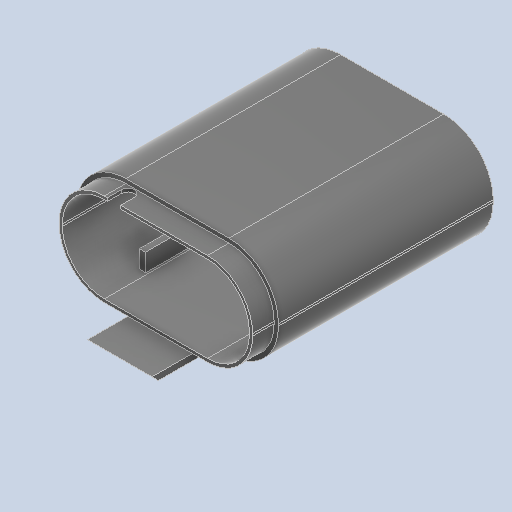
# Autodesk Inventor part: fullback
Saved by Autodesk Inventor 2024 (Build 280153000, 153)
## iProperties
Created: 2023-10-23
Part Number: fullback
Material: Acetal Resin, Black
Document SubType Name: Modeling
Designer: User Account
Density: 1.425 g/cm^3
Appearance: Smooth - Black
Author: User Account
Autodesk Inventor part; units mm, degrees
ref_plane "YZ Plane" through (0, 0, 0) normal (1, 0, 0) x (0, 1, 0)
ref_plane "XZ Plane" through (0, 0, 0) normal (0, 1, 0) x (-1, 0, 0)
ref_plane "XY Plane" through (0, 0, 0) normal (0, 0, 1) x (1, 0, 0)
sketch "Sketch1" plane through (0, 0, 0) normal (0, 0, 1) x (1, 0, 0)
  line L0 (71.0137, 43.5924) -> (23.0137, 43.5924)
  line L1 (23.0137, 41.5924) -> (71.0137, 41.5924)
  line L2 (71.0137, -1.4076) -> (23.0137, -1.4076)
  line L3 (23.0137, -3.4076) -> (71.0137, -3.4076)
  line L4 (2.0137, 19.5924) -> (2.0137, 20.5924)
  arc A0 (23.0137, 41.5924) -> (2.0137, 20.5924) centre (23.0137, 20.5924) ccw
  arc A1 (2.0137, 19.5924) -> (23.0137, -1.4076) centre (23.0137, 19.5924) ccw
  arc A2 (23.0137, 43.5924) -> (0.0137, 20.5924) centre (23.0137, 20.5924) ccw
  line L5 (0.0137, 20.5924) -> (0.0137, 19.5924)
  arc A3 (0.0137, 19.5924) -> (23.0137, -3.4076) centre (23.0137, 19.5924) ccw
  arc A4 (71.0137, -1.4076) -> (92.0137, 19.5924) centre (71.0137, 19.5924) ccw
  arc A5 (71.0137, -3.4076) -> (94.0137, 19.5924) centre (71.0137, 19.5924) ccw
  line L6 (92.0137, 20.5924) -> (92.0137, 19.5924)
  line L7 (94.0137, 19.5924) -> (94.0137, 20.5924)
  arc A6 (92.0137, 20.5924) -> (71.0137, 41.5924) centre (71.0137, 20.5924) ccw
  arc A7 (94.0137, 20.5924) -> (71.0137, 43.5924) centre (71.0137, 20.5924) ccw
  line L8 (71.0137, 40.0924) -> (23.0137, 40.0924)
  arc A8 (23.0137, 40.0924) -> (3.5137, 20.5924) centre (23.0137, 20.5924) ccw
  line L9 (3.5137, 20.5924) -> (3.5137, 19.5924)
  arc A9 (3.5137, 19.5924) -> (23.0137, 0.0924) centre (23.0137, 19.5924) ccw
  line L10 (23.0137, 0.0924) -> (71.0137, 0.0924)
  arc A10 (71.0137, 0.0924) -> (90.5137, 19.5924) centre (71.0137, 19.5924) ccw
  line L11 (90.5137, 19.5924) -> (90.5137, 20.5924)
  arc A11 (90.5137, 20.5924) -> (71.0137, 40.0924) centre (71.0137, 20.5924) ccw
  line L12 (74.7637, 0.4563) -> (74.7637, 8.4563)
  line L13 (19.2637, 8.4563) -> (19.2637, 0.4563)
  line L14 (19.2637, 8.4563) -> (22.1219, 8.4563)
  line L15 (22.1219, 8.4563) -> (22.1219, -0.3887)
  line L16 (22.1219, -0.3887) -> (19.2637, -0.3887)
  line L17 (19.2637, -0.3887) -> (19.2637, 8.4563)
  line L18 (74.7637, 8.4563) -> (74.7637, 0.4563)
  line L19 (74.7637, 8.4563) -> (71.9055, 8.4563)
  line L20 (71.9055, 8.4563) -> (71.9055, -0.3887)
  line L21 (71.9055, -0.3887) -> (74.7637, -0.3887)
  line L22 (74.7637, -0.3887) -> (74.7637, 8.4563)
  point P0 (30.5866, -26.4774)
  point P1 (2.0137, 41.5924)
  point P2 (92.0137, 41.5924)
  point P3 (92.0137, -1.4076)
  point P4 (-31.8038, -33.8139)
  point P5 (2.0137, 20.0924)
  point P6 (19.2637, 0.4563)
  point P7 (71.9055, 0.1128)
  dimension "d0" = 90
  dimension "d1" = 43
  dimension "d2" = 21
  dimension "d3" = 21
  dimension "d4" = 2
  dimension "d12" = 1.5
  dimension "d13" = 55.5
  dimension "d14" = 15.75
  dimension "d15" = 15.75
  dimension "d16" = 8
  constraints: 46 end point, 25 point on circle, 12 centre point, 9 parallel, 8 tangent, 6 point on line, 4 perpendicular, 2 equal radius, 2 horizontal, 1 midpoint, 14 other
  measures "d0" distance of point (2.014, 41.592) point (92.014, 41.592)
  measures "d1" distance of point (92.014, 41.592) point (92.014, -1.408)
  measures "d2" radius of A0
  measures "d3" radius of A1
  measures "d4" distance between parallel lines of L1 L0
  measures "d12" distance between parallel lines of L1 L8
  measures "d13" distance of L12.end L13.start
  measures "d14" distance between parallel lines of L9 L13
  measures "d15" distance between parallel lines of L11 L12
  measures "d16" distance of L12.start L12.end
extrude "Extrusion1" add sketch "Sketch1" along normal blind 2 contours A7 L7 A5 L3 A3 L5 A2 L0 | L1 A6 L6 A4 L2 A1 L4 A0 | A11 L11 A10 L12 L19 L20 L10 A9 L15 L14 L13 L9 A8 L8 | L22 L21 L20 A10 | A10 L20 L19 L12 | L13 L14 L15 A9 | A9 L15 L16 L17
extrude "Extrusion2" add sketch "Sketch1" along normal blind 100 contours A7 L7 A5 L3 A3 L5 A2 L0
extrude "Extrusion3" add sketch "Sketch1" along normal blind 110 contours L1 A6 L6 A4 L2 A1 L4 A0 | L22 L21 L20 A10 | A9 L15 L16 L17
extrude "Extrusion4" add sketch "Sketch1" along normal blind 90 contours A10 L20 L19 L12 | L13 L14 L15 A9 | A9 L15 L16 L17
sketch "Sketch2" plane through (23.0137, 41.5924, 100) normal (0, 1, 0) x (1, 0, 0)
  line L0 (4.5, -16.4538) -> (4.5, -3.5462) construction
  line L1 (0, -10) -> (48, -10) projected
  line L2 (7.55, -16.4538) -> (7.55, -3.5462)
  line L3 (1.45, -3.5462) -> (1.45, -16.4538)
  arc A0 (1.45, -16.4538) -> (7.55, -16.4538) centre (4.5, -16.4538) ccw
  arc A1 (7.55, -3.5462) -> (1.45, -3.5462) centre (4.5, -3.5462) ccw
  line L4 (0, 0) -> (0, -10) projected
  point P0 (-23.0137, 100)
  point P1 (4.5, -10)
  point P2 (1.45, -10)
  point P3 (7.55, -10)
  dimension "d25" = 1.45
  dimension "d26" = 3.05
  constraints: 8 end point, 4 point on circle, 4 tangent, 2 centre point, 1 midpoint, 1 parallel, 1 perpendicular, 1 point on line
  measures "d25" distance from line of L4 L3.start
  measures "d26" distance from line of L2 L0.end
extrude "Extrusion5" cut sketch "Sketch2" against normal blind 12 contours L3 A1 L2 L1
sketch "Sketch3" plane through (23.0137, -3.4076, 0) normal (0, -1, 0) x (1, 0, 0)
  line L0 (25.5, 63) -> (22.5, 63)
  line L1 (22.5, 63) -> (22.5, 48)
  line L2 (22.5, 48) -> (25.5, 48)
  line L3 (25.5, 48) -> (25.5, 63)
  line L4 (48, 0) -> (48, 100) projected
  line L5 (0, 0) -> (0, 100) projected
  line L6 (0, 100) -> (48, 100) projected
  point P0 (-23.0137, 0)
  dimension "d29" = 15
  dimension "d30" = 3
  dimension "d31" = 22.5
  dimension "d32" = 22.5
  dimension "d33" = 37
  constraints: 8 end point, 2 parallel, 1 horizontal, 1 perpendicular
  measures "d29" distance of L2.end L0.start
  measures "d30" distance of L1.end L2.end
  measures "d31" distance between parallel lines of L4 L3
  measures "d32" distance between parallel lines of L5 L1
  measures "d33" distance between parallel lines of L6 L0
extrude "Extrusion6" add sketch "Sketch3" along normal blind 10
sketch "Sketch4" plane through (48.5137, -3.4076, 63) normal (1, 0, 0) x (0, 0, -1)
  line L0 (0, 0) -> (21.8599, 0)
  line L1 (0, 0) -> (15, 0)
  line L2 (15, 0) -> (15, -20.5)
  line L3 (0, -20.5) -> (0, 0)
  arc A0 (0, -20.5) -> (7.5, -28) centre (7.5, -20.5) ccw
  arc A1 (7.5, -28) -> (15, -20.5) centre (7.5, -20.5) ccw
  circle A2 centre (7.5, -20.5) radius 2.5
  point P0 (63, 3.4076)
  point P1 (15, -28)
  point P2 (0, -28)
  point P3 (7.5, -28)
  point P4 (15, 0)
  dimension "d40" = 28
  dimension "d41" = 15
  dimension "d42" = 7.5
  dimension "d43" = 5
  constraints: 8 end point, 4 point on circle, 3 centre point, 2 horizontal, 2 point on line, 2 tangent, 1 coincident, 1 concentric, 1 parallel, 1 perpendicular, 7 other
  measures "d40" distance of L1.end point (15, -28)
  measures "d41" distance of point (15, -28) point (0, -28)
  measures "d42" radius of A0
  measures "d43" diameter of A2
extrude "Extrusion7" add sketch "Sketch4" along normal blind 2.93
sketch "Sketch5" plane through (45.5137, -3.4076, 48) normal (-1, 0, 0) x (0, 0, 1)
  line L0 (0, 0) -> (31.1912, 0)
  line L1 (0, 0) -> (15, 0)
  line L2 (15, 0) -> (15, -20.5)
  line L3 (0, -20.5) -> (0, 0)
  arc A0 (0, -20.5) -> (7.5, -28) centre (7.5, -20.5) ccw
  arc A1 (7.5, -28) -> (15, -20.5) centre (7.5, -20.5) ccw
  circle A2 centre (7.5, -20.5) radius 2.5
  line L4 (0, 0) -> (0, -10) projected
  line L5 (0, -10) -> (15, -10)
  line L6 (15, -10) -> (15, 0)
  line L7 (15, 0) -> (0, 0)
  line L8 (0, 0) -> (0, -10)
  point P0 (-48, 3.4076)
  point P1 (15, -28)
  point P2 (0, -28)
  point P3 (15, -10)
  point P4 (15, 0)
  point P5 (7.5, -28)
  dimension "d46" = 28
  dimension "d47" = 15
  dimension "d48" = 7.5
  dimension "d49" = 5
  constraints: 16 end point, 4 point on circle, 3 centre point, 3 horizontal, 3 parallel, 2 perpendicular, 2 point on line, 2 tangent, 1 coincident, 1 concentric, 7 other
  measures "d46" distance of L1.end point (15, -28)
  measures "d47" distance of point (15, -28) point (0, -28)
  measures "d48" radius of A0
  measures "d49" diameter of A2
extrude "Extrusion8" add sketch "Sketch5" along normal blind 5.91 contours L0 L2 L5 L3
extrude "Extrusion9" add sketch "Sketch5" along normal blind 2.93 contours L5 L2 A1 A0 L3
sketch "Sketch6" plane through (51.4437, -3.4076, 63) normal (1, 0, 0) x (0, 0, -1)
  line L0 (0, -10) -> (15, -10) projected
  line L1 (15, -10) -> (0, -10)
  line L2 (0, -10) -> (0, 0)
  line L3 (0, 0) -> (15, 0)
  line L4 (15, 0) -> (15, -10)
  point P0 (63, 3.4076)
  point P1 (0, 0)
  constraints: 8 end point, 2 parallel, 1 horizontal, 1 perpendicular
extrude "Extrusion10" add sketch "Sketch6" along normal blind 2.98
sketch "Sketch7" plane through (23.0137, -3.4076, 0) normal (0, -1, 0) x (1, 0, 0)
  line L0 (39, 34.6398) -> (9, 34.6398)
  line L1 (9, 34.6398) -> (9, 126.8335)
  line L2 (9, 126.8335) -> (39, 126.8335)
  line L3 (39, 126.8335) -> (39, 34.6398)
  line L4 (48, 0) -> (48, 100) projected
  line L5 (0, 0) -> (0, 100) projected
  point P0 (-23.0137, 0)
  point P1 (48, 50)
  dimension "d56" = 9
  dimension "d57" = 9
  constraints: 8 end point, 2 parallel, 1 horizontal, 1 midpoint, 1 perpendicular
  measures "d56" distance from line of point (48, 50) L3
  measures "d57" distance between parallel lines of L5 L1
extrude "Extrusion11" add sketch "Sketch7" along normal blind 3
chamfer "Chamfer1" distance 3 angle 45 4 edges at (47.0137, -3.4076, 34.6398) (62.0137, -3.4076, 67.3199) (32.0137, -3.4076, 67.3199) (47.0137, -6.4076, 126.8335)
chamfer "Chamfer2" distance 3 angle 45 4 edges at (39.6037, -6.4076, 55.5) (47.0137, -6.4076, 63) (49.9687, -6.4076, 48) (54.4237, -6.4076, 55.5)
body "Solid1"
